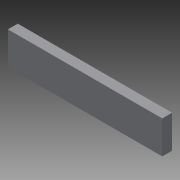
# Autodesk Inventor part: 11.75 in side
Saved by Autodesk Inventor 2015 (Build 190159000, 159)
## iProperties
Created: 2015-01-25
Part Number: 11.75 in side
Material: Generic
Document SubType Name: Modeling
Designer: Michael7
Density: 1 g/cm^3
Appearance: Default
Author: Michael7
Autodesk Inventor part; units mm, degrees
ref_plane "YZ Plane" through (0, 0, 0) normal (1, 0, 0) x (0, 1, 0)
ref_plane "XZ Plane" through (0, 0, 0) normal (0, 1, 0) x (-1, 0, 0)
ref_plane "XY Plane" through (0, 0, 0) normal (0, 0, 1) x (1, 0, 0)
sketch "Sketch1" plane through (0, 0, 0) normal (0, 0, 1) x (1, 0, 0)
  line L0 (-298.45, 63.5) -> (0, 63.5)
  line L1 (0, 63.5) -> (0, 0)
  line L2 (0, 0) -> (-298.45, 0)
  line L3 (-298.45, 0) -> (-298.45, 63.5)
  dimension "d0" = 63.5
  dimension "d1" = 298.45
  constraints: 8 end point, 2 parallel, 1 horizontal, 1 perpendicular
  measures "d0" distance of L0.end L1.end
  measures "d1" distance of L0.start L0.end
extrude "Extrusion1" add sketch "Sketch1" along normal blind 19.05
body "Solid1"
